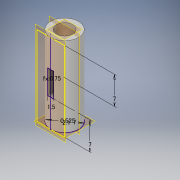
# Autodesk Inventor part: モータジョイント
Saved by Autodesk Inventor 2019.3 (Build 233278000, 278)
## iProperties
Created: 2019-08-08
Part Number: モータジョイント
Material: Generic
Document SubType Name: Modeling
Designer: ushiyama
Density: 1 g/cm^3
Appearance: Default
Author: ushiyama
Autodesk Inventor part; units mm, degrees
ref_plane "YZ Plane" through (0, 0, 0) normal (1, 0, 0) x (0, 1, 0)
sketch "スケッチ2" plane through (0, 0, 0) normal (0, 1, 0) x (-1, 0, 0)
  circle A0 centre (0, 0) radius 3.5
  dimension "d9" = 7
  constraints: 1 centre point, 1 coincident
  measures "d9" diameter of A0
sketch "スケッチ1" plane through (0, 0, 0) normal (0, 1, 0) x (-1, 0, 0)
  arc A0 (-0.525, -0.9093) -> (-0.525, 0.9093) centre (0, 0) ccw
  line L0 (-0.525, -0.9093) -> (-0.525, 0.9093)
  dimension "d0" = 2.1
  dimension "d2" = 0.525
  constraints: 2 end point, 2 point on circle, 1 centre point, 1 coincident, 1 vertical
  measures "d0" diameter of A0
  measures "d2" distance from line of point (0, 0) L0
extrude "押し出し1" add sketch "スケッチ2" along normal blind 20
extrude "押し出し2" cut sketch "スケッチ1" along normal blind 2.8
ref_plane "作業平面1" through (0, 20, 0) normal (0, 1, 0) x (1, 0, 0)
ref_plane "作業平面2" through (0, 0, 3.5) normal (0, 0, 1) x (1, 0, 0)
sketch "スケッチ4" plane through (0, 0, 3.5) normal (0, 0, 1) x (1, 0, 0)
  line L0 (3.5, 20) -> (-3.5, 20) projected
  line L1 (-3.5, 0) -> (3.5, 0) projected
  line L2 (3.5, 0) -> (3.5, 20) projected
  line L3 (-3.5, 0) -> (-3.5, 20) projected
  line L4 (-0.75, 7) -> (0.75, 7)
  line L5 (0.75, 7) -> (0.75, 13)
  line L6 (0.75, 13) -> (-0.75, 13)
  line L7 (-0.75, 13) -> (-0.75, 7)
  line L8 (0, 20) -> (0, 0)
  dimension "d14" = 7
  dimension "d15" = 7
  dimension "d16" = 1.5
  dimension "d18" = 0.75
  constraints: 10 end point, 2 parallel, 1 horizontal, 1 midpoint, 1 perpendicular, 1 vertical
  measures "d14" distance between parallel lines of L1 L4
  measures "d15" distance between parallel lines of L0 L6
  measures "d16" distance between parallel lines of L5 L7
  measures "d18" distance between parallel lines of L5 L8
extrude "押し出し4" cut sketch "スケッチ4" against normal blind 3.5 contours L8 L4 L7 L6 | L6 L5 L4 L8
sketch "スケッチ3" plane through (0, 20, 0) normal (0, 1, 0) x (1, 0, 0)
  circle A0 centre (0, 0) radius 3.5 projected
  circle A1 centre (0, 0) radius 2.05
  dimension "d11" = 4.1
  constraints: 1 centre point, 1 coincident
  measures "d11" diameter of A1
extrude "押し出し5" cut sketch "スケッチ3" against normal blind 4.2 contours A1
equation "\"d18\" = 0.5 * d16"
